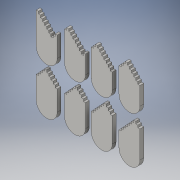
# Autodesk Inventor part: Wave_Zoetrope
Saved by Autodesk Inventor 2016 (Build 200138000, 138)
## iProperties
Created: 2018-12-05
Part Number: Wave_Zoetrope
Material: Generic
Document SubType Name: Modeling
Designer: student
Density: 1 g/cm^3
Appearance: Default
Author: student
Autodesk Inventor part; units mm, degrees
ref_plane "YZ Plane" through (0, 0, 0) normal (1, 0, 0) x (0, 1, 0)
ref_plane "XZ Plane" through (0, 0, 0) normal (0, 1, 0) x (-1, 0, 0)
ref_plane "XY Plane" through (0, 0, 0) normal (0, 0, 1) x (1, 0, 0)
sketch "Sketch1" plane through (0, 0, 0) normal (0, 0, 1) x (1, 0, 0)
  line L0 (0, 0) -> (25.4, 0)
  line L1 (25.4, 0) -> (25.4, 24.4929)
  line L2 (0, 38.1) -> (0, 0)
  line L3 (12.7, 27.2143) -> (12.7, 0)
  line L4 (0, 23.0237) -> (2.54, 23.0237) construction
  line L5 (2.54, 23.0237) -> (5.08, 23.0237) construction
  line L6 (5.08, 23.0237) -> (7.62, 23.0237) construction
  line L7 (7.62, 23.0237) -> (10.16, 23.0237) construction
  line L8 (10.16, 23.0237) -> (12.7, 23.0237) construction
  line L9 (2.54, 38.1) -> (2.54, 0)
  line L10 (5.08, 35.3786) -> (5.08, 0)
  line L11 (7.62, 32.6571) -> (7.62, 0)
  line L12 (10.16, 29.9357) -> (10.16, 0)
  line L13 (12.7, 23.0237) -> (15.24, 23.0237) construction
  line L14 (15.24, 23.0237) -> (17.78, 23.0237) construction
  line L15 (17.78, 23.0237) -> (20.32, 23.0237) construction
  line L16 (20.32, 23.0237) -> (22.86, 23.0237) construction
  line L17 (22.86, 23.0237) -> (25.4, 23.0237) construction
  line L18 (15.24, 24.4929) -> (15.24, 0)
  line L19 (17.78, 21.7714) -> (17.78, 0)
  line L20 (22.86, 24.4929) -> (22.86, 0)
  line L21 (0, 19.05) -> (-5.8932, 19.05)
  line L22 (0, 38.1) -> (-5.8932, 38.1)
  line L23 (-5.8932, 19.05) -> (-5.8932, 38.1)
  line L24 (34.3121, 0) -> (59.7121, 0)
  line L25 (59.7121, 0) -> (59.7121, 21.7714)
  line L26 (34.3121, 35.3786) -> (34.3121, 0)
  line L27 (66.7172, 0) -> (92.1172, 0)
  line L28 (92.1172, 0) -> (92.1172, 19.05)
  line L29 (66.7172, 32.6571) -> (66.7172, 0)
  line L30 (100.2453, 0) -> (125.6453, 0)
  line L31 (125.6453, 0) -> (125.6453, 21.7714)
  line L32 (100.2453, 29.9357) -> (100.2453, 0)
  line L33 (47.0121, 29.9357) -> (47.0121, 0)
  line L34 (34.3121, 21.4312) -> (36.8521, 21.4312) construction
  line L35 (36.8521, 21.4312) -> (39.3921, 21.4312) construction
  line L36 (39.3921, 21.4312) -> (41.9321, 21.4312) construction
  line L37 (41.9321, 21.4312) -> (44.4721, 21.4312) construction
  line L38 (44.4721, 21.4312) -> (47.0121, 21.4312) construction
  line L39 (47.0121, 21.4312) -> (49.5521, 21.4312) construction
  line L40 (49.5521, 21.4312) -> (52.0921, 21.4312) construction
  line L41 (52.0921, 21.4312) -> (54.6321, 21.4312) construction
  line L42 (54.6321, 21.4312) -> (57.1721, 21.4312) construction
  line L43 (57.1721, 21.4312) -> (59.7121, 21.4312) construction
  line L44 (36.8521, 38.1) -> (36.8521, 0)
  line L45 (39.3921, 38.1) -> (39.3921, 0)
  line L46 (41.9321, 35.3786) -> (41.9321, 0)
  line L47 (44.4721, 32.6571) -> (44.4721, 0)
  line L48 (49.5521, 27.2143) -> (49.5521, 0)
  line L49 (52.0921, 24.4929) -> (52.0921, 0)
  line L50 (54.6321, 21.7714) -> (54.6321, 0)
  line L51 (57.1721, 21.7714) -> (57.1721, 0)
  line L52 (-2.3979, 19.05) -> (-2.3979, 21.7714)
  line L53 (-2.3979, 21.7714) -> (-2.3979, 24.4929)
  line L54 (-2.3979, 24.4929) -> (-2.3979, 27.2143)
  line L55 (-2.3979, 27.2143) -> (-2.3979, 29.9357)
  line L56 (-2.3979, 29.9357) -> (-2.3979, 32.6571)
  line L57 (-2.3979, 32.6571) -> (-2.3979, 35.3786)
  line L58 (-2.3979, 35.3786) -> (-2.3979, 38.1)
  line L59 (2.54, 35.3786) -> (5.08, 35.3786)
  line L60 (5.08, 32.6571) -> (7.62, 32.6571)
  line L61 (7.62, 29.9357) -> (10.16, 29.9357)
  line L62 (10.16, 27.2143) -> (12.7, 27.2143)
  line L63 (12.7, 24.4929) -> (15.24, 24.4929)
  line L64 (15.24, 21.7714) -> (17.78, 21.7714)
  line L65 (17.78, 19.05) -> (20.32, 19.05)
  line L66 (20.32, 21.7714) -> (22.86, 21.7714)
  line L67 (22.86, 24.4929) -> (25.4, 24.4929)
  line L68 (36.8521, 35.3786) -> (34.3121, 35.3786)
  line L69 (39.3921, 35.3786) -> (41.9321, 35.3786)
  line L70 (41.9321, 32.6571) -> (44.4721, 32.6571)
  line L71 (44.4721, 29.9357) -> (47.0121, 29.9357)
  line L72 (47.0121, 27.2143) -> (49.5521, 27.2143)
  line L73 (49.5521, 24.4929) -> (52.0921, 24.4929)
  line L74 (52.0921, 21.7714) -> (54.6321, 21.7714)
  line L75 (54.6321, 19.05) -> (57.1721, 19.05)
  line L76 (57.1721, 21.7714) -> (59.7121, 21.7714)
  line L77 (79.4172, 32.6571) -> (79.4172, 0)
  line L78 (66.7172, 23.1321) -> (69.2572, 23.1321) construction
  line L79 (69.2572, 23.1321) -> (71.7972, 23.1321) construction
  line L80 (71.7972, 23.1321) -> (74.3372, 23.1321) construction
  line L81 (74.3372, 23.1321) -> (76.8772, 23.1321) construction
  line L82 (76.8772, 23.1321) -> (79.4172, 23.1321) construction
  line L83 (79.4172, 23.1321) -> (81.9572, 23.1321) construction
  line L84 (81.9572, 23.1321) -> (84.4972, 23.1321) construction
  line L85 (84.4972, 23.1321) -> (87.0372, 23.1321) construction
  line L86 (87.0372, 23.1321) -> (89.5772, 23.1321) construction
  line L87 (89.5772, 23.1321) -> (92.1172, 23.1321) construction
  line L88 (69.2572, 35.3786) -> (69.2572, 0)
  line L89 (71.7972, 38.1) -> (71.7972, 0)
  line L90 (74.3372, 38.1) -> (74.3372, 0)
  line L91 (76.8772, 35.3786) -> (76.8772, 0)
  line L92 (81.9572, 29.9357) -> (81.9572, 0)
  line L93 (84.4972, 27.2143) -> (84.4972, 0)
  line L94 (87.0372, 24.4929) -> (87.0372, 0)
  line L95 (89.5772, 21.7714) -> (89.5772, 0)
  line L96 (71.7972, 35.3786) -> (69.2572, 35.3786)
  line L97 (69.2572, 32.6571) -> (66.7172, 32.6571)
  line L98 (74.3372, 35.3786) -> (76.8772, 35.3786)
  line L99 (76.8772, 32.6571) -> (79.4172, 32.6571)
  line L100 (79.4172, 29.9357) -> (81.9572, 29.9357)
  line L101 (81.9572, 27.2143) -> (84.4972, 27.2143)
  line L102 (84.4972, 24.4929) -> (87.0372, 24.4929)
  line L103 (87.0372, 21.7714) -> (89.5772, 21.7714)
  line L104 (89.5772, 19.05) -> (92.1172, 19.05)
  line L105 (112.9453, 35.3786) -> (112.9453, 0)
  line L106 (100.2453, 23.1321) -> (102.7853, 23.1321) construction
  line L107 (102.7853, 23.1321) -> (105.3253, 23.1321) construction
  line L108 (105.3253, 23.1321) -> (107.8653, 23.1321) construction
  line L109 (107.8653, 23.1321) -> (110.4053, 23.1321) construction
  line L110 (110.4053, 23.1321) -> (112.9453, 23.1321) construction
  line L111 (112.9453, 23.1321) -> (115.4853, 23.1321) construction
  line L112 (115.4853, 23.1321) -> (118.0253, 23.1321) construction
  line L113 (118.0253, 23.1321) -> (120.5653, 23.1321) construction
  line L114 (120.5653, 23.1321) -> (123.1053, 23.1321) construction
  line L115 (123.1053, 23.1321) -> (125.6453, 23.1321) construction
  line L116 (102.7853, 32.6571) -> (102.7853, 0)
  line L117 (105.3253, 35.3786) -> (105.3253, 0)
  line L118 (107.8653, 38.1) -> (107.8653, 0)
  line L119 (110.4053, 38.1) -> (110.4053, 0)
  line L120 (115.4853, 32.6571) -> (115.4853, 0)
  line L121 (118.0253, 29.9357) -> (118.0253, 0)
  line L122 (120.5653, 27.2143) -> (120.5653, 0)
  line L123 (123.1053, 24.4929) -> (123.1053, 0)
  line L124 (107.8653, 35.3786) -> (105.3253, 35.3786)
  line L125 (105.3253, 32.6571) -> (102.7853, 32.6571)
  line L126 (102.7853, 29.9357) -> (100.2453, 29.9357)
  line L127 (110.4053, 35.3786) -> (112.9453, 35.3786)
  line L128 (112.9453, 32.6571) -> (115.4853, 32.6571)
  line L129 (115.4853, 29.9357) -> (118.0253, 29.9357)
  line L130 (118.0253, 27.2143) -> (120.5653, 27.2143)
  line L131 (120.5653, 24.4929) -> (123.1053, 24.4929)
  line L132 (123.1053, 21.7714) -> (125.6453, 21.7714)
  line L133 (36.8521, 38.1) -> (39.3921, 38.1)
  line L134 (71.7972, 38.1) -> (74.3372, 38.1)
  line L135 (107.8653, 38.1) -> (110.4053, 38.1)
  line L136 (0, 38.1) -> (2.54, 38.1)
  line L137 (20.32, 21.7714) -> (20.32, 0)
  arc A0 (0, 0) -> (25.4, 0) centre (12.7, 0) ccw
  arc A1 (34.3121, 0) -> (59.7121, 0) centre (47.0121, 0) ccw
  arc A2 (66.7172, 0) -> (92.1172, 0) centre (79.4172, 0) ccw
  arc A3 (100.2453, 0) -> (125.6453, 0) centre (112.9453, 0) ccw
  line L138 (25.4, -31.9465) -> (25.4, -56.4393)
  line L139 (25.4, -56.4393) -> (0, -56.4393)
  line L140 (0, -56.4393) -> (0, -18.3393)
  line L141 (59.7121, -29.2251) -> (59.7121, -56.4393)
  line L142 (59.7121, -56.4393) -> (34.3121, -56.4393)
  line L143 (34.3121, -56.4393) -> (34.3121, -31.9465)
  line L144 (92.1172, -26.5036) -> (92.1172, -56.4393)
  line L145 (92.1172, -56.4393) -> (66.7172, -56.4393)
  line L146 (66.7172, -56.4393) -> (66.7172, -34.6679)
  line L147 (125.6453, -23.7822) -> (125.6453, -56.4393)
  line L148 (125.6453, -56.4393) -> (100.2453, -56.4393)
  line L149 (100.2453, -56.4393) -> (100.2453, -37.3893)
  line L150 (2.54, -26.5036) -> (2.54, -56.4393)
  line L151 (5.08, -23.7822) -> (5.08, -56.4393)
  line L152 (7.62, -21.0608) -> (7.62, -56.4393)
  line L153 (10.16, -18.3393) -> (10.16, -56.4393)
  line L154 (12.7, -18.3393) -> (12.7, -56.4393)
  line L155 (15.24, -56.4393) -> (15.24, -21.0608)
  line L156 (17.78, -23.7822) -> (17.78, -56.4393)
  line L157 (20.32, -26.5036) -> (20.32, -56.4393)
  line L158 (22.86, -29.2251) -> (22.86, -56.4393)
  line L159 (0, -37.3893) -> (-5.8932, -37.3893)
  line L160 (-5.8932, -37.3893) -> (-5.8932, -18.3393)
  line L161 (-5.8932, -18.3393) -> (0, -18.3393)
  line L162 (-2.9466, -37.3893) -> (-2.9466, -34.6679)
  line L163 (-2.9466, -34.6679) -> (-2.9466, -31.9465)
  line L164 (-2.9466, -31.9465) -> (-2.9466, -29.2251)
  line L165 (-2.9466, -29.2251) -> (-2.9466, -26.5036)
  line L166 (-2.9466, -26.5036) -> (-2.9466, -23.7822)
  line L167 (-2.9466, -23.7822) -> (-2.9466, -21.0608)
  line L168 (-2.9466, -21.0608) -> (-2.9466, -18.3393)
  line L169 (10.16, -21.0608) -> (7.62, -21.0608)
  line L170 (7.62, -23.7822) -> (5.08, -23.7822)
  line L171 (5.08, -26.5036) -> (2.54, -26.5036)
  line L172 (2.54, -29.2251) -> (0, -29.2251)
  line L173 (12.7, -21.0608) -> (15.24, -21.0608)
  line L174 (15.24, -23.7822) -> (17.78, -23.7822)
  line L175 (17.78, -26.5036) -> (20.32, -26.5036)
  line L176 (20.32, -29.2251) -> (22.86, -29.2251)
  line L177 (22.86, -31.9465) -> (25.4, -31.9465)
  line L178 (47.0121, -18.3393) -> (47.0121, -56.4393)
  line L179 (36.8521, -29.2251) -> (36.8521, -56.4393)
  line L180 (39.3921, -26.5036) -> (39.3921, -56.4393)
  line L181 (41.9321, -23.7822) -> (41.9321, -56.4393)
  line L182 (44.4721, -21.0608) -> (44.4721, -56.4393)
  line L183 (49.5521, -18.3393) -> (49.5521, -56.4393)
  line L184 (52.0921, -21.0608) -> (52.0921, -56.4393)
  line L185 (54.6321, -23.7822) -> (54.6321, -56.4393)
  line L186 (57.1721, -26.5036) -> (57.1721, -56.4393)
  line L187 (47.0121, -21.0608) -> (44.4721, -21.0608)
  line L188 (49.5521, -21.0608) -> (52.0921, -21.0608)
  line L189 (44.4721, -23.7822) -> (41.9321, -23.7822)
  line L190 (52.0921, -23.7822) -> (54.6321, -23.7822)
  line L191 (41.9321, -26.5036) -> (39.3921, -26.5036)
  line L192 (54.6321, -26.5036) -> (57.1721, -26.5036)
  line L193 (39.3921, -29.2251) -> (36.8521, -29.2251)
  line L194 (57.1721, -29.2251) -> (59.7121, -29.2251)
  line L195 (36.8521, -31.9465) -> (34.3121, -31.9465)
  line L196 (79.4172, -21.0608) -> (79.4172, -56.4393)
  line L197 (69.2572, -31.9465) -> (69.2572, -56.4393)
  line L198 (71.7972, -29.2251) -> (71.7972, -56.4393)
  line L199 (74.3372, -26.5036) -> (74.3372, -56.4393)
  line L200 (76.8772, -23.7822) -> (76.8772, -56.4393)
  line L201 (81.9572, -18.3393) -> (81.9572, -56.4393)
  line L202 (84.4972, -18.3393) -> (84.4972, -56.4393)
  line L203 (87.0372, -21.0608) -> (87.0372, -56.4393)
  line L204 (89.5772, -23.7822) -> (89.5772, -56.4393)
  line L205 (81.9572, -21.0608) -> (79.4172, -21.0608)
  line L206 (84.4972, -21.0608) -> (87.0372, -21.0608)
  line L207 (87.0372, -23.7822) -> (89.5772, -23.7822)
  line L208 (89.5772, -26.5036) -> (92.1172, -26.5036)
  line L209 (79.4172, -23.7822) -> (76.8772, -23.7822)
  line L210 (76.8772, -26.5036) -> (74.3372, -26.5036)
  line L211 (74.3372, -29.2251) -> (71.7972, -29.2251)
  line L212 (71.7972, -31.9465) -> (69.2572, -31.9465)
  line L213 (69.2572, -34.6679) -> (66.7172, -34.6679)
  line L214 (112.9453, -23.7822) -> (112.9453, -56.4393)
  line L215 (102.7853, -34.6679) -> (102.7853, -56.4393)
  line L216 (105.3253, -31.9465) -> (105.3253, -56.4393)
  line L217 (107.8653, -29.2251) -> (107.8653, -56.4393)
  line L218 (110.4053, -26.5036) -> (110.4053, -56.4393)
  line L219 (115.4853, -21.0608) -> (115.4853, -56.4393)
  line L220 (118.0253, -18.3393) -> (118.0253, -56.4393)
  line L221 (120.5653, -18.3393) -> (120.5653, -56.4393)
  line L222 (123.1053, -21.0608) -> (123.1053, -56.4393)
  line L223 (118.0253, -21.0608) -> (115.4853, -21.0608)
  line L224 (120.5653, -21.0608) -> (123.1053, -21.0608)
  line L225 (123.1053, -23.7822) -> (125.6453, -23.7822)
  line L226 (115.4853, -23.7822) -> (112.9453, -23.7822)
  line L227 (112.9453, -26.5036) -> (110.4053, -26.5036)
  line L228 (110.4053, -29.2251) -> (107.8653, -29.2251)
  line L229 (107.8653, -31.9465) -> (105.3253, -31.9465)
  line L230 (105.3253, -34.6679) -> (102.7853, -34.6679)
  line L231 (102.7853, -37.3893) -> (100.2453, -37.3893)
  line L232 (10.16, -18.3393) -> (12.7, -18.3393)
  line L233 (47.0121, -18.3393) -> (49.5521, -18.3393)
  line L234 (81.9572, -18.3393) -> (84.4972, -18.3393)
  line L235 (118.0253, -18.3393) -> (120.5653, -18.3393)
  arc A4 (0, -56.4393) -> (25.4, -56.4393) centre (12.7, -56.4393) ccw
  arc A5 (34.3121, -56.4393) -> (59.7121, -56.4393) centre (47.0121, -56.4393) ccw
  arc A6 (66.7172, -56.4393) -> (92.1172, -56.4393) centre (79.4172, -56.4393) ccw
  arc A7 (100.2453, -56.4393) -> (125.6453, -56.4393) centre (112.9453, -56.4393) ccw
  dimension "d2" = 2.54
  dimension "d3" = 2.54
  dimension "d4" = 2.54
  dimension "d5" = 2.54
  dimension "d6" = 2.54
  dimension "d7" = 2.54
  dimension "d8" = 2.54
  dimension "d9" = 2.54
  dimension "d20" = 2.54
  dimension "d21" = 2.54
  dimension "d22" = 2.54
  dimension "d23" = 2.54
  dimension "d24" = 2.54
  dimension "d25" = 2.54
  dimension "d26" = 2.54
  dimension "d27" = 2.54
  dimension "d28" = 2.7214
  dimension "d29" = 2.7214
  dimension "d30" = 2.7214
  dimension "d31" = 2.7214
  dimension "d32" = 2.7214
  dimension "d33" = 2.7214
  dimension "d34" = 2.54
  dimension "d35" = 2.54
  dimension "d36" = 2.54
  dimension "d37" = 2.54
  dimension "d38" = 2.54
  dimension "d39" = 2.54
  dimension "d40" = 2.54
  dimension "d41" = 2.54
  dimension "d42" = 2.54
  dimension "d43" = 2.54
  dimension "d44" = 2.54
  dimension "d45" = 2.54
  dimension "d46" = 2.54
  dimension "d47" = 2.54
  dimension "d48" = 2.54
  dimension "d49" = 2.54
  dimension "d50" = 2.54
  dimension "d51" = 2.54
  dimension "d52" = 2.54
  dimension "d53" = 2.54
  dimension "d59" = 2.7214
  dimension "d60" = 2.7214
  dimension "d61" = 2.7214
  dimension "d62" = 2.7214
  dimension "d63" = 2.7214
  dimension "d64" = 2.7214
  dimension "d65" = 2.7214
  constraints: 456 end point, 180 point on line, 61 vertical, 36 perpendicular, 30 parallel, 21 horizontal, 16 point on circle, 14 tangent, 8 centre point, 4 midpoint, 1 coincident, 98 other
  measures "d2" distance of L4.start L4.end
  measures "d3" distance of L4.end L5.end
  measures "d4" distance of L5.end L6.end
  measures "d5" distance of L6.end L7.end
  measures "d6" distance of L8.end L13.end
  measures "d7" distance of L14.end L13.end
  measures "d8" distance of L14.end L15.end
  measures "d9" distance of L15.end L16.end
  measures "d20" distance of L34.start L34.end
  measures "d21" distance of L34.end L35.end
  measures "d22" distance of L35.end L36.end
  measures "d23" distance of L36.end L37.end
  measures "d24" distance of L38.end L39.end
  measures "d25" distance of L39.end L40.end
  measures "d26" distance of L40.end L41.end
  measures "d27" distance of L41.end L42.end
  measures "d28" distance of L52.start L52.end
  measures "d29" distance of L52.end L53.end
  measures "d30" distance of L53.end L54.end
  measures "d31" distance of L54.end L55.end
  measures "d32" distance of L55.end L56.end
  measures "d33" distance of L56.end L57.end
  measures "d34" distance of L78.start L78.end
  measures "d35" distance of L78.end L79.end
  measures "d36" distance of L79.end L80.end
  measures "d37" distance of L80.end L81.end
  measures "d38" distance of L81.end L82.end
  measures "d39" distance of L82.end L83.end
  measures "d40" distance of L83.end L84.end
  measures "d41" distance of L84.end L85.end
  measures "d42" distance of L86.end L85.end
  measures "d43" distance of L86.end L87.end
  measures "d44" distance of L106.start L106.end
  measures "d45" distance of L106.end L107.end
  measures "d46" distance of L107.end L108.end
  measures "d47" distance of L108.end L109.end
  measures "d48" distance of L109.end L110.end
  measures "d49" distance of L110.end L111.end
  measures "d50" distance of L111.end L112.end
  measures "d51" distance of L112.end L113.end
  measures "d52" distance of L113.end L114.end
  measures "d53" distance of L115.end L114.end
  measures "d59" distance of L162.start L162.end
  measures "d60" distance of L162.end L163.end
  measures "d61" distance of L163.end L164.end
  measures "d62" distance of L164.end L165.end
  measures "d63" distance of L165.end L166.end
  measures "d64" distance of L166.end L167.end
  measures "d65" distance of L167.end L168.end
extrude "Extrusion1" add sketch "Sketch1" along normal blind 4.572 contours L2 L136 L9 L0 | L0 A0 | L9 L59 L10 L0 | L0 L20 L67 L1 | L10 L60 L11 L0 | L0 L137 L66 L20 | L11 L61 L12 L0 | L0 L19 L65 L137 | L12 L62 L3 L0 | L0 L18 L64 L19 | L3 L63 L18 L0 | L26 L68 L44 L24 | L24 A1 | L44 L133 L45 L24 | L24 L51 L76 L25 | L45 L69 L46 L24 | L24 L50 L75 L51 | L46 L70 L47 L24 | L24 L49 L74 L50 | L47 L71 L33 L24 | L24 L48 L73 L49 | L33 L72 L48 L24 | L29 L97 L88 L27 | L27 A2 | L88 L96 L89 L27 | L27 L95 L104 L28 | L89 L134 L90 L27 | L27 L94 L103 L95 | L90 L98 L91 L27 | L27 L93 L102 L94 | L91 L99 L77 L27 | L27 L92 L101 L93 | L77 L100 L92 L27 | L32 L126 L116 L30 | L30 A3 | L116 L125 L117 L30 | L30 L123 L132 L31 | L117 L124 L118 L30 | L30 L122 L131 L123 | L118 L135 L119 L30 | L30 L121 L130 L122 | L119 L127 L105 L30 | L30 L120 L129 L121 | L105 L128 L120 L30 | L138 L139 L158 L177 | A4 L139 | L158 L139 L157 L176 | L140 L172 L150 L139 | L139 L156 L175 L157 | L150 L171 L151 L139 | L139 L155 L174 L156 | L151 L170 L152 L139 | L139 L154 L173 L155 | L152 L169 L153 L139 | L139 L153 L232 L154 | L141 L142 L186 L194 | A5 L142 | L186 L142 L185 L192 | L143 L195 L179 L142 | L142 L184 L190 L185 | L179 L193 L180 L142 | L142 L183 L188 L184 | L180 L191 L181 L142 | L142 L178 L233 L183 | L181 L189 L182 L142 | L142 L182 L187 L178 | L144 L145 L204 L208 | A6 L145 | L204 L145 L203 L207 | L146 L213 L197 L145 | L145 L202 L206 L203 | L197 L212 L198 L145 | L145 L201 L234 L202 | L198 L211 L199 L145 | L145 L196 L205 L201 | L199 L210 L200 L145 | L145 L200 L209 L196 | L147 L148 L222 L225 | A7 L148 | L222 L148 L221 L224 | L149 L231 L215 L148 | L148 L220 L235 L221 | L215 L230 L216 L148 | L148 L219 L223 L220 | L216 L229 L217 L148 | L148 L214 L226 L219 | L217 L228 L218 L148 | L148 L218 L227 L214
body "Solid1"
